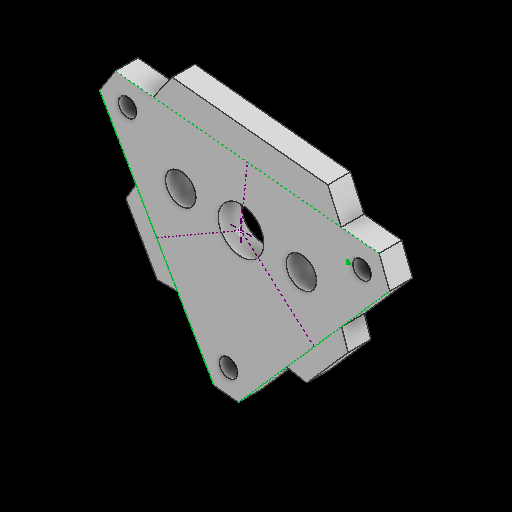
# Autodesk Inventor part: TongueMount
Saved by Autodesk Inventor 2025.2 (Build 292293000, 293)
## iProperties
Created: 2024-12-18
Part Number: TongueMount
Material: Generic
Document SubType Name: Sheet Metal
Designer: valer
Density: 1 g/cm^3
Appearance: Default
Sheet Metal Rule: Default
Flat Pattern Width: 3.17746 cm
Flat Pattern Length: 3.8505 cm
Flat Pattern Area: 12.2348 cm^2
Sheet Metal Width: 31.775 mm
Sheet Metal Length: 38.505 mm
Sheet Metal Area: 1223.478 mm^2
Author: valer
Autodesk Inventor part; units mm, degrees
ref_plane "YZ Plane" through (0, 0, 0) normal (1, 0, 0) x (0, 1, 0)
ref_plane "XZ Plane" through (0, 0, 0) normal (0, 1, 0) x (-1, 0, 0)
ref_plane "XY Plane" through (0, 0, 0) normal (0, 0, 1) x (1, 0, 0)
sketch "Sketch1" plane through (0, 0, 0) normal (0, 0, 1) x (1, 0, 0)
  circle A0 centre (-29.1799, 3.0736) radius 3.175 construction
  circle A1 centre (1.7526, 0) radius 3.175 construction
  circle A2 centre (-15.8567, -20.0304) radius 3.175 construction
  circle A3 centre (-29.1799, 3.0736) radius 1.2
  circle A4 centre (1.7526, 0) radius 1.2
  circle A5 centre (-15.8567, -20.0304) radius 1.2
  line L0 (-29.1799, 3.0736) -> (1.7526, 0) construction
  line L1 (-13.7137, 1.5368) -> (-15.8567, -20.0304) construction
  line L2 (-30.7954, 6.4247) -> (3.9959, 2.9677)
  line L3 (3.9959, 2.9677) -> (5.4173, -0.6401)
  line L4 (5.4173, -0.6401) -> (-14.5484, -23.3511)
  line L5 (-14.5484, -23.3511) -> (-17.7927, -23.0287)
  line L6 (-17.7927, -23.0287) -> (-32.899, 3.1671)
  line L7 (-32.899, 3.1671) -> (-30.7954, 6.4247)
  point P0 (0, 0)
  point P1 (-16.1706, -23.1899)
  point P2 (-31.8472, 4.7959)
  dimension "d0" = 2.4
  dimension "d1" = 2.4
  dimension "d2" = 2.4
  constraints: 16 end point, 3 centre point, 3 coincident, 3 midpoint, 2 tangent, 1 parallel, 10 other
  measures "d0" diameter of A3
  measures "d1" diameter of A4
  measures "d2" diameter of A5
extrude "Plate1" add sketch "Sketch1" along normal blind 3
sketch "Sketch2" plane through (0, 0, 3) normal (0, 0, 1) x (1, 0, 0)
  line L0 (-17.7927, -23.0287) -> (-32.899, 3.1671) construction
  line L1 (-30.7954, 6.4247) -> (3.9959, 2.9677) construction
  line L2 (5.4173, -0.6401) -> (-14.5484, -23.3511) construction
  line L3 (-17.7927, -23.0287) -> (-32.899, 3.1671) construction
  line L4 (-25.3459, -9.9308) -> (-14.2154, -3.5122) construction
  line L5 (-14.2154, -3.5122) -> (-13.3997, 4.6962) construction
  line L6 (-14.2154, -3.5122) -> (-4.5656, -11.9956) construction
  line L7 (5.4173, -0.6401) -> (-14.5484, -23.3511) construction
  point P0 (0, 0)
  constraints: 6 end point, 3 midpoint, 3 perpendicular, 1 coincident
sketch "Sketch3" plane through (0, 0, 3) normal (0, 0, 1) x (1, 0, 0)
  arc A0 (-5.0898, -2.6774) -> (-6.5829, -2.3304) centre (-6.2546, -4.3032) ccw projected
  arc A1 (-6.5829, -2.3304) -> (-5.0898, -2.6774) centre (-6.2546, -4.3032) ccw projected
  arc A2 (-21.0113, -1.0954) -> (-22.5045, -0.7484) centre (-22.1762, -2.7212) ccw projected
  arc A3 (-22.5045, -0.7484) -> (-21.0113, -1.0954) centre (-22.1762, -2.7212) ccw projected
  circle A4 centre (-14.2154, -3.5122) radius 3 projected
extrude "Extrusion1" cut sketch "Sketch3" against normal through all
sketch "Sketch4" plane through (0, 0, 0) normal (0, 0, -1) x (-1, 0, 0)
  line L0 (30.7954, 6.4247) -> (-3.9959, 2.9677) projected
  line L1 (0.9857, 3.4627) -> (2.77, 7.4096)
  line L2 (2.77, 7.4096) -> (13.0288, 8.429)
  line L3 (13.0288, 8.429) -> (13.3997, 4.6962) construction
  arc A0 (9.3955, 4.3921) -> (1.4831, 3.2621) centre (5.4635, 3.6576) ccw construction
  line L4 (25.8137, 5.9297) -> (23.2877, 9.4483)
  line L5 (23.2877, 9.4483) -> (13.0288, 8.429)
  line L6 (-5.4173, -0.6401) -> (14.5484, -23.3511) projected
  line L7 (0.9442, -7.8763) -> (0.0881, -10.4082)
  line L8 (0.0881, -10.4082) -> (2.8272, -13.5239)
  line L9 (2.8272, -13.5239) -> (4.5656, -11.9956) construction
  line L10 (-5.4173, -0.6401) -> (14.5484, -23.3511) projected
  arc A1 (3.0652, -12.6595) -> (11.0452, -12.2104) centre (7.0456, -12.264) ccw construction
  line L11 (8.1869, -16.1149) -> (5.5662, -16.6395)
  line L12 (5.5662, -16.6395) -> (2.8272, -13.5239)
  line L13 (17.7927, -23.0287) -> (32.899, 3.1671) projected
  line L14 (28.0858, -5.1794) -> (29.4234, -7.4934)
  line L15 (29.4234, -7.4934) -> (27.351, -11.0871)
  line L16 (25.2786, -14.6808) -> (27.351, -11.0871)
  line L17 (22.6059, -14.6822) -> (25.2786, -14.6808)
  point P0 (0, 0)
  dimension "d6" = 120
  dimension "d7" = 120
  constraints: 28 end point, 9 symmetric about line, 4 tangent, 2 midpoint, 2 parallel, 2 perpendicular, 2 point on line
  measures "d6" angle of L0 L1
  measures "d7" angle of L6 L7
extrude "Extrusion2" add sketch "Sketch4" against normal up to surface (3 mm away)
equation "\"d3\" = Thickness"
equation "\"BendRadius\" = Thickness"
equation "\"BendReliefWidth\" = Thickness"
equation "\"BendReliefDepth\" = 0.5 * Thickness"
equation "\"CornerReliefSize\" = 4 * Thickness"
equation "\"MinimumRemnant\" = 2 * Thickness"
equation "\"TransitionRadius\" = BendRadius"
equation "\"JacobiRadiusSize\" = BendRadius"
equation "\"GapSize\" = Thickness"
equation "\"Thickness\" = 3"
body "Solid1"
